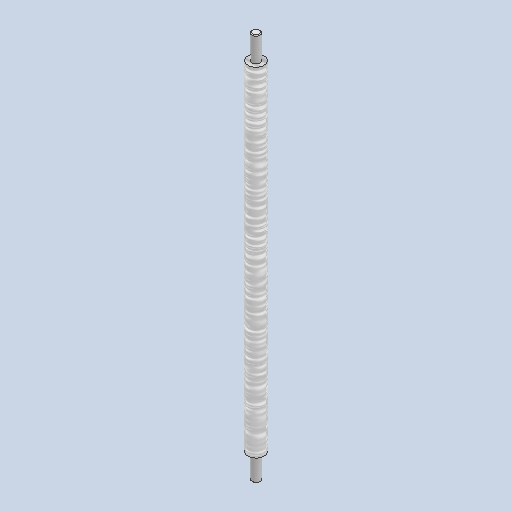
# Autodesk Inventor part: Columnas
Saved by Autodesk Inventor 2025.3 (Build 293356030, 356C)
## iProperties
Created: 2024-12-23
Part Number: Columnas
Material: Aluminum 7075
Document SubType Name: Modeling
Designer: Usuario
Density: 2.81 g/cm^3
Appearance: Satin - Brushed Heavy
Author: Usuario
Autodesk Inventor part; units mm, degrees
ref_plane "YZ Plane" through (0, 0, 0) normal (1, 0, 0) x (0, 1, 0)
ref_plane "XZ Plane" through (0, 0, 0) normal (0, 1, 0) x (-1, 0, 0)
ref_plane "XY Plane" through (0, 0, 0) normal (0, 0, 1) x (1, 0, 0)
sketch "Boceto1" plane through (0, 0, 0) normal (0, 0, 1) x (1, 0, 0)
  line L0 (0, -70.5) -> (0, 70.5)
  line L1 (0, 70.5) -> (-1.5, 70.5)
  line L2 (-1.5, 70.5) -> (-1.5, 61.5)
  line L3 (-1.5, 61.5) -> (-3, 61.5)
  line L4 (-3, 61.5) -> (-3, -61.5)
  line L5 (-3, -61.5) -> (-1.5, -61.5)
  line L6 (-1.5, -61.5) -> (-1.5, -70.5)
  line L7 (-1.5, -70.5) -> (0, -70.5)
  point P0 (0, 0)
  point P1 (0, 0)
  dimension "d1" = 3
  dimension "d2" = 6
  dimension "d3" = 9
  dimension "d4" = 123
  dimension "d8" = 9
  constraints: 16 end point, 5 perpendicular, 2 point on line, 1 coincident, 1 horizontal, 1 midpoint, 1 vertical
  measures "d1" diameter of L2 L0
  measures "d2" diameter of L4 L0
  measures "d3" distance of L1.end L2.end
  measures "d4" distance of L3.end L4.end
  measures "d8" distance of L5.end L6.end
revolve "Revolución1" add sketch "Boceto1" angle 360 about axis through (0, -70.5, 0) along (0, 1, 0)
thread "Rosca1" size "M3x0.5" class "6g" standard "ANSI Metric M Profile" full length
chamfer "Chaflán1" distance 0.3067 angle 45 2 edges at (1.5, 70.5, 0) (1.5, -70.5, 0)
